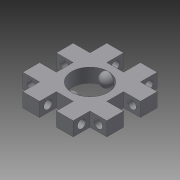
# Autodesk Inventor part: crossCenterMini
Saved by Autodesk Inventor 2015 (Build 190159000, 159)
## iProperties
Created: 2016-10-15
Part Number: crossCenterMini
Material: Generic
Document SubType Name: Modeling
Designer: Bardo91
Density: 1 g/cm^3
Appearance: Default
Author: Bardo91
Autodesk Inventor part; units mm, degrees
ref_plane "YZ Plane" through (0, 0, 0) normal (1, 0, 0) x (0, 1, 0)
ref_plane "XZ Plane" through (0, 0, 0) normal (0, 1, 0) x (-1, 0, 0)
ref_plane "XY Plane" through (0, 0, 0) normal (0, 0, 1) x (1, 0, 0)
sketch "Sketch1" plane through (0, 0, 0) normal (0, 0, 1) x (1, 0, 0)
  line L0 (0, 0) -> (0, 6)
  line L1 (0, 6) -> (6, 6)
  line L2 (6, 6) -> (6, 0)
  line L3 (6, 0) -> (12, 0)
  line L4 (12, 0) -> (12, 6)
  line L5 (12, 6) -> (18, 6)
  line L6 (18, 6) -> (18, 0)
  line L7 (18, 0) -> (24, 0)
  line L8 (24, 0) -> (24, -6)
  line L9 (24, -6) -> (18, -6)
  line L10 (18, -6) -> (18, -12)
  line L11 (18, -12) -> (24, -12)
  line L12 (24, -12) -> (24, -18)
  line L13 (24, -18) -> (18, -18)
  line L14 (18, -18) -> (18, -24)
  line L15 (18, -24) -> (12, -24)
  line L16 (12, -24) -> (12, -18)
  line L17 (12, -18) -> (6, -18)
  line L18 (6, -18) -> (6, -24)
  line L19 (6, -24) -> (0, -24)
  line L20 (0, -24) -> (0, -18)
  line L21 (0, -18) -> (-6, -18)
  line L22 (-6, -18) -> (-6, -12)
  line L23 (-6, -12) -> (0, -12)
  line L24 (0, -12) -> (0, -6)
  line L25 (0, -6) -> (-6, -6)
  line L26 (-6, -6) -> (-6, 0)
  line L27 (-6, 0) -> (0, 0)
  dimension "d55" = 6
  dimension "d56" = 6
  dimension "d57" = 6
  dimension "d58" = 6
  dimension "d59" = 6
  dimension "d60" = 6
  dimension "d61" = 6
  dimension "d62" = 90
  dimension "d63" = 6
  dimension "d64" = 6
  dimension "d65" = 90
  dimension "d66" = 6
  dimension "d67" = 6
  dimension "d68" = 6
  dimension "d69" = 6
  dimension "d70" = 6
  dimension "d71" = 6
  dimension "d72" = 6
  dimension "d73" = 6
  dimension "d74" = 6
  dimension "d75" = 6
  dimension "d76" = 6
  dimension "d77" = 90
  constraints: 56 end point, 15 perpendicular, 13 point on line, 3 horizontal, 2 vertical
  measures "d55" distance of L0.start L0.end
  measures "d56" distance of L0.end L1.end
  measures "d57" distance of L2.end L3.end
  measures "d58" distance of L3.end L4.end
  measures "d59" distance of L4.end L5.end
  measures "d60" distance of L6.end L7.end
  measures "d61" distance of L7.end L8.end
  measures "d62" angle of L7 L8
  measures "d63" distance of L8.end L9.end
  measures "d64" distance of L9.end L10.end
  measures "d65" angle of L10 L9
  measures "d66" distance of L10.end L11.end
  measures "d67" distance of L11.end L12.end
  measures "d68" distance of L13.end L14.end
  measures "d69" distance of L14.end L15.end
  measures "d70" distance of L16.end L17.end
  measures "d71" distance of L18.end L19.end
  measures "d72" distance of L19.end L20.end
  measures "d73" distance of L20.end L21.end
  measures "d74" distance of L21.end L22.end
  measures "d75" distance of L23.end L24.end
  measures "d76" distance of L24.end L25.end
  measures "d77" angle of L25 L24
extrude "Extrusion1" add sketch "Sketch1" along normal blind 5
sketch "Sketch6" plane through (0, 0, 5) normal (0, 0, 1) x (1, 0, 0)
  line L0 (12, 0) -> (6, 0)
  line L1 (9, 0) -> (9, -18)
  line L2 (6, -18) -> (12, -18)
  line L3 (18, -12) -> (18, -6)
  line L4 (18, -9) -> (9, -9)
  arc A0 (6.546663, -2.980769) -> (11.453337, -2.980769) centre (9, -2.5) ccw
  arc A1 (11.453337, -15.019231) -> (6.546663, -15.019231) centre (9, -15.5) ccw
  arc A2 (6.546663, -2.980769) -> (9, -15.5) centre (9, -9) ccw
  arc A3 (11.453337, -15.019231) -> (11.453337, -2.980769) centre (9, -9) ccw
  point P0 (0, 0)
  dimension "d79" = 5
  dimension "d80" = 5
  constraints: 9 point on circle, 4 centre point, 4 end point, 4 midpoint, 2 point on line, 1 coincident
  measures "d79" diameter of A0
  measures "d80" diameter of A1
extrude "Extrusion6" cut sketch "Sketch6" against normal through all contours A0 A3 L4 L1 | L1 A1 A2 A0 | L4 A3 A1 L1
sketch "Sketch7" plane through (-6, -18, 0) normal (0, -1, 0) x (1, 0, 0)
  line L0 (0, 0) -> (0, 2.5)
  line L1 (0, 0) -> (0, 5) projected
  line L2 (0, 2.5) -> (3, 2.5)
  circle A0 centre (3, 2.5) radius 1.5
  point P0 (6, 0)
  dimension "d83" = 3
  dimension "d84" = 3
  constraints: 4 end point, 1 centre point, 1 coincident, 1 horizontal, 1 midpoint
  measures "d83" distance of L0.end L2.end
  measures "d84" diameter of A0
extrude "Extrusion7" cut sketch "Sketch7" against normal through all
pattern_circular "Circular Pattern3" count 4 over 360 about axis through (9, -9, 5) along (0, 0, -1) of "Extrusion7"
fillet "Fillet2" radius 2.47 4 edges at (9, -5, 5) (9, -5, 0) (9, -13, 5) (9, -13, 0)
body "Solid1"
